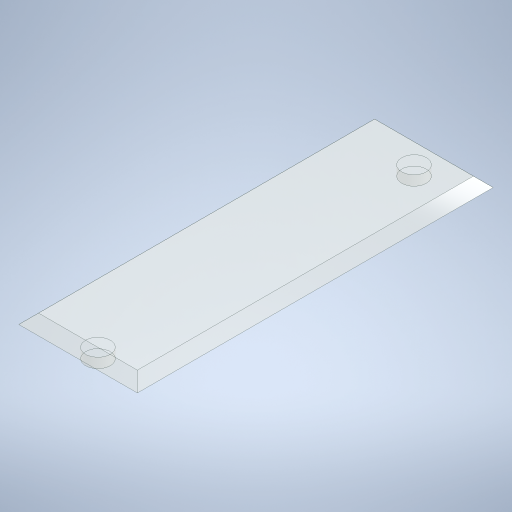
# Autodesk Inventor part: TerminalBlockLid
Saved by Autodesk Inventor 2024 (Build 280153000, 153)
## iProperties
Created: 2023-06-18
Part Number: TerminalBlockLid
Material: Generic
Document SubType Name: Modeling
Designer: 18179
Density: 1 g/cm^3
Appearance: Clear
Author: 18179
Autodesk Inventor part; units mm, degrees
ref_plane "YZ Plane" through (0, 0, 0) normal (1, 0, 0) x (0, 1, 0)
ref_plane "XZ Plane" through (0, 0, 0) normal (0, 1, 0) x (-1, 0, 0)
ref_plane "XY Plane" through (0, 0, 0) normal (0, 0, 1) x (1, 0, 0)
sketch "Sketch1" plane through (0, 0, 0) normal (0, 1, 0) x (-1, 0, 0)
  line L0 (-21.4179, -39.4841) -> (-21.4179, -33.3379)
  line L1 (-21.4179, -33.3379) -> (-13.4169, -33.3379)
  line L2 (-13.4169, -33.3379) -> (-13.4169, -39.4841)
  line L3 (-13.4169, -39.4841) -> (-21.4179, -39.4841)
  line L4 (-21.4179, 41.7458) -> (-21.4179, 47.8919)
  line L5 (-21.4179, 47.8919) -> (-13.4169, 47.8919)
  line L6 (-13.4169, 47.8919) -> (-13.4169, 41.7458)
  line L7 (-13.4169, 41.7458) -> (-21.4179, 41.7458)
  circle A0 centre (-26.6249, -36.411) radius 3.175
  circle A1 centre (-26.6249, 44.8188) radius 3.175
  line L8 (-31.8319, 47.8919) -> (-31.8319, 41.7458)
  line L9 (-31.8319, 41.7458) -> (-39.8329, 41.7458)
  line L10 (-39.8329, 41.7458) -> (-39.8329, 47.8919)
  line L11 (-39.8329, 47.8919) -> (-31.8319, 47.8919)
  line L12 (-31.8319, -33.3379) -> (-31.8319, -39.4841)
  line L13 (-31.8319, -39.4841) -> (-39.8329, -39.4841)
  line L14 (-39.8329, -39.4841) -> (-39.8329, -33.3379)
  line L15 (-39.8329, -33.3379) -> (-31.8319, -33.3379)
  line L16 (-41.8649, 3.1879) -> (-27.6409, 3.1879)
  line L17 (-27.6409, 3.1879) -> (-27.6409, -6.9721)
  line L18 (-27.6409, -6.9721) -> (-41.8649, -6.9721)
  line L19 (-41.8649, -6.9721) -> (-41.8649, -9.0041)
  line L20 (-41.8649, -9.0041) -> (-27.6409, -9.0041)
  line L21 (-27.6409, -9.0041) -> (-27.6409, -19.1641)
  line L22 (-27.6409, -19.1641) -> (-41.8649, -19.1641)
  line L23 (-41.8649, -19.1641) -> (-41.8649, -21.1961)
  line L24 (-41.8649, -21.1961) -> (-27.6409, -21.1961)
  line L25 (-27.6409, -21.1961) -> (-27.6409, -31.3561)
  line L26 (-27.6409, -31.3561) -> (-41.8649, -31.3561)
  line L27 (-41.8649, -31.3561) -> (-41.8649, -41.5161)
  line L28 (-41.8649, -41.5161) -> (-11.3849, -41.5161)
  line L29 (-11.3849, -41.5161) -> (-11.3849, -31.3561)
  line L30 (-11.3849, -31.3561) -> (-25.6089, -31.3561)
  line L31 (-25.6089, -31.3561) -> (-25.6089, -21.1961)
  line L32 (-25.6089, -21.1961) -> (-11.3849, -21.1961)
  line L33 (-11.3849, -21.1961) -> (-11.3849, -19.1641)
  line L34 (-11.3849, -19.1641) -> (-25.6089, -19.1641)
  line L35 (-25.6089, -19.1641) -> (-25.6089, -9.0041)
  line L36 (-25.6089, -9.0041) -> (-11.3849, -9.0041)
  line L37 (-11.3849, -9.0041) -> (-11.3849, -6.9721)
  line L38 (-11.3849, -6.9721) -> (-25.6089, -6.9721)
  line L39 (-25.6089, -6.9721) -> (-25.6089, 3.1879)
  line L40 (-25.6089, 3.1879) -> (-11.3849, 3.1879)
  line L41 (-11.3849, 3.1879) -> (-11.3849, 5.2199)
  line L42 (-11.3849, 5.2199) -> (-25.6089, 5.2199)
  line L43 (-25.6089, 5.2199) -> (-25.6089, 15.3799)
  line L44 (-25.6089, 15.3799) -> (-11.3849, 15.3799)
  line L45 (-11.3849, 15.3799) -> (-11.3849, 17.4119)
  line L46 (-11.3849, 17.4119) -> (-25.6089, 17.4119)
  line L47 (-25.6089, 17.4119) -> (-25.6089, 27.5719)
  line L48 (-25.6089, 27.5719) -> (-11.3849, 27.5719)
  line L49 (-11.3849, 27.5719) -> (-11.3849, 29.6039)
  line L50 (-11.3849, 29.6039) -> (-25.6089, 29.6039)
  line L51 (-25.6089, 29.6039) -> (-25.6089, 39.7639)
  line L52 (-25.6089, 39.7639) -> (-11.3849, 39.7639)
  line L53 (-11.3849, 39.7639) -> (-11.3849, 49.9239)
  line L54 (-11.3849, 49.9239) -> (-41.8649, 49.9239)
  line L55 (-41.8649, 49.9239) -> (-41.8649, 39.7639)
  line L56 (-41.8649, 39.7639) -> (-27.6409, 39.7639)
  line L57 (-27.6409, 39.7639) -> (-27.6409, 29.6039)
  line L58 (-27.6409, 29.6039) -> (-41.8649, 29.6039)
  line L59 (-41.8649, 29.6039) -> (-41.8649, 27.5719)
  line L60 (-41.8649, 27.5719) -> (-27.6409, 27.5719)
  line L61 (-27.6409, 27.5719) -> (-27.6409, 17.4119)
  line L62 (-27.6409, 17.4119) -> (-41.8649, 17.4119)
  line L63 (-41.8649, 17.4119) -> (-41.8649, 15.3799)
  line L64 (-41.8649, 15.3799) -> (-27.6409, 15.3799)
  line L65 (-27.6409, 15.3799) -> (-27.6409, 5.2199)
  line L66 (-27.6409, 5.2199) -> (-41.8649, 5.2199)
  line L67 (-41.8649, 5.2199) -> (-41.8649, 3.1879)
  line L68 (-11.3849, -31.3561) -> (-11.3849, 39.7639)
  line L69 (-41.8649, 39.7639) -> (-41.8649, -31.3561)
  point P0 (0, 0)
  constraints: 140 end point, 2 centre point, 1 collinear, 1 parallel
extrude "Extrusion1" add sketch "Sketch1" along normal blind 2.54 contours L0 L1 L2 L3 | L4 L5 L6 L7 | L8 L9 L10 L11 | L12 L13 L14 L15 | L67 L66 L65 L64 L63 L62 L61 L60 L59 L58 L57 L56 L55 L54 L53 L52 L51 L50 L49 L48 L47 L46 L45 L44 L43 L42 L41 L40 L39 L38 L37 L36 L35 L34 L33 L32 L31 L30 L29 L28 L27 L26 L25 L24 L23 L22 L21 L20 L19 L18 L17 L16 | L16 L17 L18 L69 | L69 L64 L65 L66 | L20 L21 L22 L69 | L69 L60 L61 L62 | L24 L25 L26 L69 | L69 L56 L57 L58 | L30 L31 L32 L68 | L68 L50 L51 L52 | L34 L35 L36 L68 | L68 L46 L47 L48 | L38 L39 L40 L68 | L68 L42 L43 L44
chamfer "Chamfer1" distance 2.54 angle 45 4 edges at (26.6249, 2.54, 49.9239) (41.8649, 2.54, -20.1801) (11.3849, 2.54, -36.4361) (26.6249, 2.54, -41.5161)
sketch "Sketch2" plane through (0, 0, 0) normal (0, -1, 0) x (1, 0, 0)
  circle A0 centre (26.6249, 44.8188) radius 3.175 projected
  circle A1 centre (26.6249, 44.8188) radius 3.175
  circle A2 centre (26.6249, -36.411) radius 3.175 projected
  circle A3 centre (26.6249, -36.411) radius 3.175
  point P0 (0, 0)
  constraints: 2 centre point, 2 coincident
extrude "Extrusion2" add sketch "Sketch2" along normal blind 2.54
sketch "Sketch3" plane through (26.6249, 0, 44.8188) normal (0, 1, 0) x (1, 0, 0)
  circle A0 centre (0, 81.2298) radius 3.175 projected
  circle A1 centre (0, 0) radius 3.175 projected
  point P0 (-26.6249, 44.8188)
extrude "Extrusion3" add sketch "Sketch3" along normal blind 2.54
sketch "Sketch4" plane through (11.3849, 0, 49.9239) normal (0, 0.7071068, 0.7071068) x (1, 0, 0)
  line L0 (10.0398, 1.9622) -> (22.6044, 1.9622)
  line L1 (22.6044, 1.9622) -> (22.6044, 6.858)
  line L2 (22.6044, 6.858) -> (10.0398, 6.858)
  line L3 (10.0398, 6.858) -> (10.0398, 1.9622)
  point P0 (-11.3849, 35.3015)
  constraints: 8 end point, 2 parallel, 1 horizontal, 1 perpendicular
extrude "Extrusion4" cut sketch "Sketch4" along normal blind 2.54
sketch "Sketch5" plane through (41.8649, 0, -41.5161) normal (0, 0.7071068, -0.7071068) x (-1, 0, 0)
  line L0 (9.9656, 2.1621) -> (20.0479, 2.1621)
  line L1 (20.0479, 2.1621) -> (20.0479, 4.6266)
  line L2 (20.0479, 4.6266) -> (9.9656, 4.6266)
  line L3 (9.9656, 4.6266) -> (9.9656, 2.1621)
  point P0 (41.8649, 29.3563)
  constraints: 8 end point, 2 parallel, 1 horizontal, 1 perpendicular
extrude "Extrusion5" cut sketch "Sketch5" along normal blind 2.54
body "Solid1"
